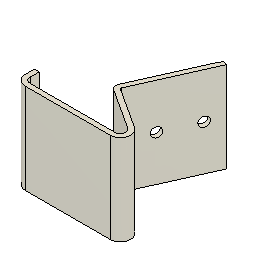
fluke101_asm (Autodesk Fusion 360 archive; units mm, degrees)
design "multimeterTiltBracketFluke101"
Autodesk Fusion 360 part; units mm, degrees
sketch "Sketch1" plane through (0, 0, 0) normal (0, 1, 0) x (1, 0, 0)
  arc A0 (31.1232, 52.6914) -> (20.5609, 48.637) centre (27.8693, 45.3831) ccw
  line L0 (31.1232, 52.6914) -> (40.2587, 48.6241)
  arc A1 (28.2837, -48.2895) -> (32.9132, -32.6608) centre (28.2837, -39.7895) ccw
  line L1 (28.2837, -48.2895) -> (-42.2163, -48.2895)
  arc A2 (-4.6567, -8.0029) -> (-2.8122, -14.2299) centre (-0.089, -10.0365) ccw
  line L2 (22.8004, 52.0184) -> (38.6317, 44.9699)
  line L3 (-46.7163, -32.2895) -> (-50.7163, -32.2895)
  line L4 (35.3386, -39.0053) -> (-23.3345, -39.0053) construction
  arc A3 (28.2837, -44.2895) -> (30.7346, -36.0155) centre (28.2837, -39.7895) ccw
  line L5 (40.2587, 48.6241) -> (38.6317, 44.9699)
  line L6 (30.7346, -36.0155) -> (-2.8122, -14.2299)
  line L7 (-50.7163, -39.7895) -> (-50.7163, -32.2895)
  line L8 (32.9132, -32.6608) -> (-0.6336, -10.8752)
  arc A4 (-46.7163, -39.7895) -> (-42.2163, -44.2895) centre (-42.2163, -39.7895) ccw
  arc A5 (-50.7163, -39.7895) -> (-42.2163, -48.2895) centre (-42.2163, -39.7895) ccw
  line L9 (-4.6567, -8.0029) -> (20.5609, 48.637)
  line L10 (28.2837, -44.2895) -> (-42.2163, -44.2895)
  line L11 (-46.7163, -39.7895) -> (-46.7163, -32.2895)
  arc A6 (22.8004, 52.0184) -> (27.1963, 53.7059) centre (27.8693, 45.3831) ccw
  arc A7 (-1.0025, -9.6298) -> (-0.6336, -10.8752) centre (-0.089, -10.0365) ccw
  line L12 (-1.0025, -9.6298) -> (27.1963, 53.7059)
  point P0 (35.3386, -39.0053)
  point P1 (-46.7163, -44.2895)
  point P2 (23.8148, 55.9453)
  dimension "d1" = 33
  dimension "d2" = 66
  dimension "d3" = 4.5
  dimension "d4" = 5
  dimension "d5" = 12
  dimension "d6" = 18
  dimension "d10" = 75
  dimension "d11" = 70
  dimension "d12" = 40
  dimension "d13" = 8
  dimension "d14" = 4.5
  constraint coincident P0 L4.start
  constraint coincident P0 L6
  constraint tangent A3 L10
  constraint tangent A3 L6
  constraint tangent A2 L6
  constraint tangent A2 L9
  constraint perpendicular L10 L11
  constraint perpendicular L0 L9
  constraint coincident P2 L9
  constraint coincident P2 L0
  constraint tangent A0 L9
  constraint tangent A0 L0
  constraint coincident P1 L10
  constraint coincident P1 L11
  constraint tangent A4 L10
  constraint tangent A4 L11
  constraint concentric A4 A5
  constraint concentric A1 A3
  constraint concentric A2 A7
  constraint concentric A0 A6
  constraint tangent L7 A5
  constraint tangent A1 L8
  constraint tangent L1 A5
  constraint tangent A1 L1
  constraint tangent L8 A7
  constraint tangent A7 L12
  measures "d1" angle of L4 L6
  measures "d2" angle of L4 L9
  measures "d3" radius of A3
  measures "d4" radius of A2
  measures "d5" distance of P1 L3.start
  measures "d6" distance of P2 L0.end
  measures "d10" distance of P1 A3.start
  measures "d11" distance of A2.start P2
  measures "d12" distance of A3.end A2.end
  measures "d13" radius of A0
  measures "d14" radius of A4
extrude "Extrude1" add sketch "Sketch1" along normal blind 75 contours A0 L2 L9 A6 L12 | A1 L1 A2 L3 A3 L6 L7 L8 A4 A5 L9 L10 L11 A6 A7 L12
sketch "Sketch2" plane through (-0.9127, 0, -0.4064) normal (-0.913545, 0, -0.406737) x (-0.406737, 0, 0.913545)
  line L0 (-52.795, 0) -> (9.205, 0)
  line L1 (9.205, 0) -> (9.205, 75)
  line L2 (9.205, 75) -> (-52.795, 75)
  line L3 (-52.795, 75) -> (-52.795, 0)
  circle A0 centre (-42.795, 37.5) radius 4
  circle A1 centre (-12.795, 37.5) radius 4
  line L4 (-31.6238, 0) -> (-31.6238, 75)
  line L5 (9.205, 37.5) -> (-64.6996, 37.5)
  dimension "d17" = 8
  dimension "d18" = 8
  dimension "d23" = 10
  dimension "d24" = 30
  constraint coincident L0 L4.start
  constraint coincident L2 L4.end
  constraint perpendicular L2 L4
  constraint perpendicular L4 L5
  constraint coincident L1 L5.start
  constraint coincident A0.centre L5
  constraint coincident A1.centre L5
  measures "d17" diameter of A0
  measures "d18" diameter of A1
  measures "d23" distance of L3 A0.centre
  measures "d24" distance of A0.centre A1.centre
extrude "Extrude2" cut sketch "Sketch2" along normal blind 18 and the other way blind 25 contours A0 L5 | A0 L5 | A1 L5 | A1 L5

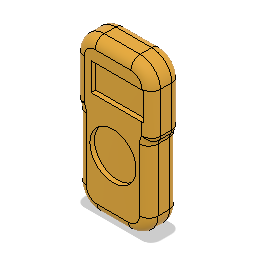
design "fluke101"
Autodesk Fusion 360 part; units mm, degrees
sketch "Sketch1" plane through (0, 0, 0) normal (0, 0, 1) x (1, 0, 0)
  line L0 (31, 65.5) -> (-31, 65.5)
  line L1 (-31, 65.5) -> (-31, -65.5)
  line L2 (-31, -65.5) -> (31, -65.5)
  line L3 (31, -65.5) -> (31, 65.5)
  line L4 (31, 65.5) -> (-31, -65.5) construction
  line L5 (-31, 65.5) -> (31, -65.5) construction
  line L6 (-31, 65.5) -> (-33, 65.5)
  line L7 (-33, 65.5) -> (-33, 10.5)
  line L8 (-33, 10.5) -> (-31, 10.5)
  line L9 (31, 10.5) -> (33, 10.5)
  line L10 (33, 10.5) -> (33, 65.5)
  line L11 (33, 65.5) -> (31, 65.5)
  line L12 (26, 47.5) -> (-19, 47.5)
  line L13 (-19, 47.5) -> (-19, 23.5)
  line L14 (-19, 23.5) -> (26, 23.5)
  line L15 (26, 23.5) -> (26, 47.5)
  line L16 (26, 47.5) -> (-19, 23.5) construction
  line L17 (-19, 47.5) -> (26, 23.5) construction
  circle A0 centre (0, -14.5) radius 20
  point P0 (3.5, 35.5)
  dimension "d1" = 62
  dimension "d2" = 131
  dimension "d3" = 2
  dimension "d4" = 2
  dimension "d6" = 76
  dimension "d7" = 76
  dimension "d16" = 45
  dimension "d17" = 24
  dimension "d18" = 18
  dimension "d19" = 40
  dimension "d20" = 80
  constraint horizontal L0
  constraint perpendicular L0 L1
  constraint parallel L0 L2
  constraint parallel L1 L3
  constraint coincident L4 origin
  constraint coincident L5 origin
  constraint perpendicular L1 L6
  constraint perpendicular L6 L7
  constraint coincident L1 L8.end
  constraint perpendicular L1 L8
  constraint coincident L3 L9.start
  constraint perpendicular L3 L9
  constraint perpendicular L0 L10
  constraint perpendicular L3 L11
  constraint horizontal L12
  constraint perpendicular L12 L13
  constraint parallel L12 L14
  constraint parallel L13 L15
  constraint coincident L16 P0
  constraint coincident L17 P0
  measures "d1" distance of L1.end L2.end
  measures "d2" distance of L0.end L1.end
  measures "d3" distance of L1 L7
  measures "d4" distance of L3 L10
  measures "d6" vertical distance of L1.end L7.end
  measures "d7" vertical distance of L2.end L9.end
  measures "d16" distance of L13.end L14.end
  measures "d17" distance of L12.end L13.end
  measures "d18" distance of L0 L12
  measures "d19" diameter of A0
  measures "d20" distance of L0 A0.centre
extrude "Extrude1" add sketch "Sketch1" against normal blind 26 contours L0 L1 L2 L3 | L3 L9 L10 L11 | L1 L6 L7 L8 | L12 L13 L14 L15 | A0
fillet "Fillet1" radius 6 4 edges at (31, 10.5, -13) (-31, 10.5, -13) (-33, 10.5, -13) (33, 10.5, -13)
fillet "Fillet2" radius 8 20 edges at (0, 65.5, 0) (-33, 39.0806, 0) (-32.7446, 10.9291, 0) (-31.2554, 7.7599, 0) (-31, -29.7361, 0) (31, -29.7361, 0) (31.2554, 7.7599, 0) (32.7446, 10.9291, 0) (33, 39.0806, 0) (0, -65.5, 0) (0, -65.5, -26) (33, 39.0806, -26) (32.7446, 10.9291, -26) (31.2554, 7.7599, -26) (31, -29.7361, -26) (-31, -29.7361, -26) (-31.2554, 7.7599, -26) (-32.7446, 10.9291, -26) (-33, 39.0806, -26) (0, 65.5, -26)
fillet "Fillet3" radius 17.5 12 edges at (30.6569, 63.1569, -2.3431) (33, 65.5, -13) (30.6569, 63.1569, -23.6569) (-30.6569, 63.1569, -23.6569) (-33, 65.5, -13) (-30.6569, 63.1569, -2.3431) (-28.6569, -63.1569, -2.3431) (-31, -65.5, -13) (-28.6569, -63.1569, -23.6569) (28.6569, -63.1569, -2.3431) (31, -65.5, -13) (28.6569, -63.1569, -23.6569)
extrude "Extrude2" cut sketch "Sketch1" against normal blind 4 contours L12 L13 L14 L15 | A0
